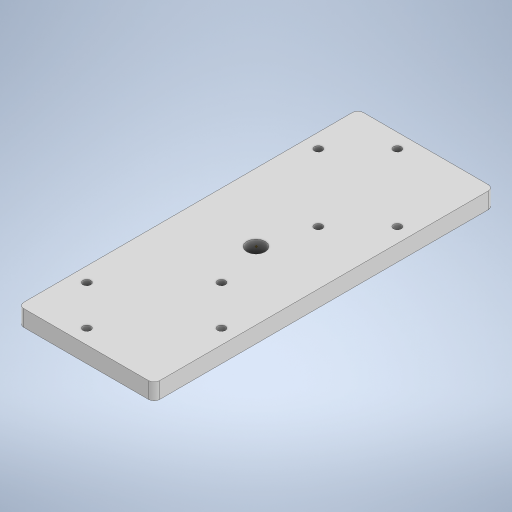
# Autodesk Inventor part: ShuttleValveShelf
Saved by Autodesk Inventor 2023 (Build 270158000, 158)
## iProperties
Created: 2023-07-21
Part Number: ShuttleValveShelf
Material: Generic
Document SubType Name: Modeling
Designer: User
Density: 1 g/cm^3
Appearance: Default
Author: User
Autodesk Inventor part; units mm, degrees
ref_plane "YZ Plane" through (0, 0, 0) normal (1, 0, 0) x (0, 1, 0)
ref_plane "XZ Plane" through (0, 0, 0) normal (0, 1, 0) x (-1, 0, 0)
ref_plane "XY Plane" through (0, 0, 0) normal (0, 0, 1) x (1, 0, 0)
sketch "Sketch1" plane through (0, 0, 0) normal (0, 1, 0) x (-1, 0, 0)
  line L0 (-25, 62.5) -> (25, 62.5)
  line L1 (25, 62.5) -> (25, -62.5)
  line L2 (25, -62.5) -> (-25, -62.5)
  line L3 (-25, -62.5) -> (-25, 62.5)
  line L4 (-25, 62.5) -> (25, -62.5) construction
  line L5 (25, 62.5) -> (-25, -62.5) construction
  point P0 (0, 0)
  dimension "d0" = 125
  dimension "d1" = 50
  constraints: 12 end point, 2 midpoint, 2 parallel, 1 horizontal, 1 perpendicular
  measures "d0" distance of L0.end L1.end
  measures "d1" distance of L0.start L0.end
extrude "Extrusion1" add sketch "Sketch1" along normal blind 6
sketch "Sketch3" plane through (0, 6, 0) normal (0, 1, 0) x (1, 0, 0)
  line L0 (25, 62.5) -> (-25, 62.5) projected
  line L1 (-25, -62.5) -> (25, -62.5) projected
  line L2 (-19.6668, -42.6187) -> (-5.1187, -57.1668)
  line L3 (-5.1187, -57.1668) -> (19.6668, -32.3813)
  line L4 (19.6668, -32.3813) -> (5.1187, -17.8332)
  line L5 (5.1187, -17.8332) -> (-19.6668, -42.6187)
  line L6 (25, -62.5) -> (25, 62.5) projected
  line L7 (-25, 62.5) -> (-25, -62.5) projected
  line L8 (5.1187, 17.8332) -> (19.6668, 32.3813)
  line L9 (19.6668, 32.3813) -> (-5.1187, 57.1668)
  line L10 (-5.1187, 57.1668) -> (-19.6668, 42.6187)
  line L11 (-19.6668, 42.6187) -> (5.1187, 17.8332)
  circle A0 centre (-19.6668, -42.6187) radius 1.45
  circle A1 centre (5.1187, -17.8332) radius 1.45
  circle A2 centre (19.6668, -32.3813) radius 1.45
  circle A3 centre (-5.1187, -57.1668) radius 1.45
  circle A4 centre (-19.6668, 42.6187) radius 1.45
  circle A5 centre (-5.1187, 57.1668) radius 1.45
  circle A6 centre (19.6668, 32.3813) radius 1.45
  circle A7 centre (5.1187, 17.8332) radius 1.45
  point P0 (0, 0)
  point P1 (0, -37.5)
  point P2 (0, 37.5)
  point P3 (0, -62.5)
  point P4 (0, 62.5)
  dimension "d5" = 125
  dimension "d7" = 35.052
  dimension "d8" = 20.574
  dimension "d9" = 50
  dimension "d10" = 10.287
  dimension "d11" = 17.526
  dimension "d12" = 35.052
  dimension "d13" = 20.574
  dimension "d14" = 17.526
  dimension "d15" = 10.287
  dimension "d16" = 2.9
  dimension "d17" = 2.9
  dimension "d18" = 2.9
  dimension "d19" = 2.9
  dimension "d20" = 2.9
  dimension "d21" = 2.9
  dimension "d22" = 2.9
  dimension "d23" = 2.9
  dimension "d24" = 25
  dimension "d25" = 25
  constraints: 16 end point, 8 centre point, 8 coincident, 4 parallel, 2 midpoint, 2 perpendicular
  measures "d5" distance between parallel lines of L0 L1
  measures "d7" distance of L2.end L3.end
  measures "d8" distance of L2.start L2.end
  measures "d9" distance between parallel lines of L6 L7
  measures "d10" distance from line of point (0, -37.5) L5
  measures "d11" distance from line of L2 point (0, -37.5)
  measures "d12" distance of L8.end L9.end
  measures "d13" distance of L8.start L8.end
  measures "d14" distance from line of point (0, 37.5) L10
  measures "d15" distance from line of L11 point (0, 37.5)
  measures "d16" diameter of A0
  measures "d17" diameter of A1
  measures "d18" diameter of A2
  measures "d19" diameter of A3
  measures "d20" diameter of A4
  measures "d21" diameter of A5
  measures "d22" diameter of A6
  measures "d23" diameter of A7
  measures "d24" distance of point (0, -62.5) point (0, -37.5)
  measures "d25" distance of point (0, 62.5) point (0, 37.5)
extrude "Extrusion2" cut sketch "Sketch3" against normal through all contours L5 A0 L2 | L2 A0 L5 | A3 L3 L2 | L2 L3 A3 | A1 L4 L5 | L5 L4 A1 | A2 L4 L3 | L3 L4 A2 | L11 A7 L8 | L8 A7 L11 | A6 L9 L8 | L8 L9 A6 | A4 L10 L11 | L11 L10 A4 | A5 L10 L9 | L9 L10 A5
hole "Hole1" at (0, 6, 0) direction (0, -1, 0) diameter 6.756 end through all clearance for "Hex Head Bolt" size "1/4" standard "Ansi Unified Screw Threads"
fillet "Fillet1" radius 2 4 edges at (25, 3, 62.5) (25, 3, -62.5) (-25, 3, -62.5) (-25, 3, 62.5)
equation "\"d10\" = 0.5 * d8"
equation "\"d11\" = 0.5 * d7"
equation "\"d14\" = 0.5 * d12"
equation "\"d15\" = 0.5 * d13"
body "Solid1"
